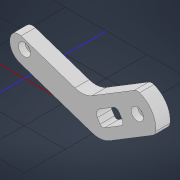
# Autodesk Inventor part: swing_arm_lg_a
Saved by Autodesk Inventor 2022.2 (Build 262287010, 287A)
## iProperties
Created: 2022-03-19
Part Number: swing_arm_lg_a
Material: Generisch
Document SubType Name: Modeling
Designer: sleib
Density: 1 g/cm^3
Appearance: Vorgabe
Author: sleib
Autodesk Inventor part; units mm, degrees
ref_plane "YZ Plane" through (0, 0, 0) normal (1, 0, 0) x (0, 1, 0)
ref_plane "XZ Plane" through (0, 0, 0) normal (0, 1, 0) x (-1, 0, 0)
ref_plane "XY Plane" through (0, 0, 0) normal (0, 0, 1) x (1, 0, 0)
sketch "Skizze1" plane through (40.1841, 0.5218, 7) normal (0, 0, 1) x (1, 0, 0)
  circle A0 centre (-33.0364, 18.6853) radius 1.7
  circle A1 centre (21.9664, 19.0079) radius 1.7
  line L0 (-34.7098, 23.5764) -> (-8.489, 14.7348)
  line L1 (-0.0887, 15.672) -> (20.4797, 28.2103)
  line L2 (29.5016, 13.8004) -> (8.4002, 0.9372)
  line L3 (-35.321, 11.9101) -> (0, 0)
  arc A2 (-8.489, 14.7348) -> (-0.0887, 15.672) centre (-5.2938, 24.2106) ccw
  arc A3 (-34.7098, 23.5764) -> (-39.7357, 21.1838) centre (-35.9878, 19.786) ccw
  arc A4 (-39.7357, 21.1838) -> (-35.321, 11.9101) centre (-33.0364, 18.6853) ccw
  arc A5 (23.0623, 28.4696) -> (20.4797, 28.2103) centre (22.0412, 25.6487) ccw
  arc A6 (29.5016, 13.8004) -> (30.9275, 16.0873) centre (27.9401, 16.362) ccw
  arc A7 (0, 0) -> (8.4002, 0.9372) centre (3.1952, 9.4758) ccw
  arc A8 (30.9275, 16.0873) -> (23.0623, 28.4696) centre (18.9779, 17.1861) ccw
  line L4 (-33.0364, 18.6853) -> (2.0366, 6.8588) construction
  line L5 (2.0366, 6.8588) -> (21.9664, 19.0079) construction
  circle A9 centre (-33.0364, 18.6853) radius 3
  circle A10 centre (21.9664, 19.0079) radius 3
  line L6 (0.9406, 10.2898) -> (4.5841, 4.3127)
  line L7 (4.5841, 4.3127) -> (15.6843, 11.0793)
  line L8 (15.6843, 11.0793) -> (12.0407, 17.0563)
  line L9 (12.0407, 17.0563) -> (0.9406, 10.2898)
  arc A11 (3.8033, 5.5935) -> (5.8649, 5.0935) centre (5.0841, 6.3743) ccw
  arc A12 (3.5022, 11.8513) -> (2.5021, 7.7282) centre (5.0637, 9.2897) ccw
  arc A13 (13.0818, 15.3486) -> (10.333, 16.0153) centre (11.374, 14.3076) ccw
  arc A14 (13.9766, 10.0383) -> (14.6433, 12.787) centre (12.9355, 11.746) ccw
  point P0 (-40.1841, -0.5218)
  dimension "d0" = 10
  dimension "d1" = 7.15
  dimension "d2" = 4
  dimension "d4" = 12
  dimension "d6" = 10
  dimension "d7" = 3.4
  dimension "d8" = 3.4
  dimension "d9" = 130
  dimension "d10" = 17
  dimension "d11" = 3.5
  dimension "d12" = 3
  dimension "d13" = 3
  dimension "d14" = 11.25
  dimension "d17" = 6
  dimension "d18" = 6
  dimension "d21" = 7
  dimension "d22" = 13
  dimension "d23" = 1.5
  dimension "d24" = 3
  dimension "d25" = 2
  dimension "d26" = 2
  dimension "d27" = 0.85
  constraints: 22 point on circle, 20 end point, 19 tangent, 15 centre point, 9 point on line, 7 parallel, 3 coincident, 1 perpendicular, 4 other
  measures "d0" radius of A7
  measures "d1" radius of A4
  measures "d2" radius of A3
  measures "d4" radius of A8
  measures "d6" radius of A2
  measures "d7" diameter of A0
  measures "d8" diameter of A1
  measures "d9" angle of L5 L4
  measures "d10" distance between parallel lines of L2 L1
  measures "d11" distance of L5.end A8.centre
  measures "d12" radius of A5
  measures "d13" radius of A6
  measures "d14" distance between parallel lines of L3 L0
  measures "d17" diameter of A9
  measures "d18" diameter of A10
  measures "d21" distance between parallel lines of L7 L9
  measures "d22" distance between parallel lines of L8 L6
  measures "d23" radius of A11
  measures "d24" radius of A12
  measures "d25" radius of A13
  measures "d26" radius of A14
  measures "d27" distance from line of L6 L4.end
extrude "Extrusion1" add sketch "Skizze1" against normal blind 7 contours L0 A2 L1 A5 A8 A6 L2 A7 L3 A4 A3 | A9 | A10 | L9 A12 L6 | A11 L7 L6 | L9 L8 A13 | A14 L8 L7
extrude "Extrusion2" cut sketch "Skizze1" against normal blind 3.2 contours A9 | A10
